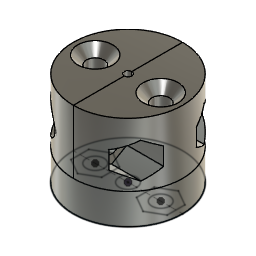
electromagnet-gripper (Autodesk Fusion 360 design; units mm, degrees)
Autodesk Fusion 360 part; units mm, degrees
note: some values were not read from the file. Chosen so that the rebuilt part matches the saved one: which bodies a step acts on; which sketch regions a step uses; which face or edge a step refers to.
sketch "Sketch1" plane through (0, 0, 0) normal (0, 0, 1) x (1, 0, 0)
sketch "Sketch1 (2)" plane through (0, 0, 0) normal (0, 0, 1) x (1, 0, 0) in component "bottom"
  circle A0 centre (0, 0) radius 12.5
  circle A1 centre (0, 0) radius 2
  circle A2 centre (-7.5, 0) radius 2
  circle A3 centre (7.5, 0) radius 2
  line L0 (0, 0) -> (12.5, 0) construction
  line L1 (0, 0) -> (-12.5, 0) construction
  line L2 (11, 2.0207) -> (7.5, 4.0415)
  line L3 (7.5, 4.0415) -> (4, 2.0207)
  line L4 (4, 2.0207) -> (4, -2.0207)
  line L5 (4, -2.0207) -> (7.5, -4.0415)
  line L6 (7.5, -4.0415) -> (11, -2.0207)
  line L7 (11, -2.0207) -> (11, 2.0207)
  line L8 (-11, -2.0207) -> (-7.5, -4.0415)
  line L9 (-7.5, -4.0415) -> (-4, -2.0207)
  line L10 (-4, -2.0207) -> (-4, 2.0207)
  line L11 (-4, 2.0207) -> (-7.5, 4.0415)
  line L12 (-7.5, 4.0415) -> (-11, 2.0207)
  line L13 (-11, 2.0207) -> (-11, -2.0207)
  point P0 (7.5, 0)
  point P1 (-7.5, 0)
  dimension "d1" = 25
  dimension "d2" = 4
  dimension "d3" = 4
  dimension "d4" = 3.5
  dimension "d6" = 5
  dimension "d7" = 5
  constraint coincident A0.centre A1.centre
  constraint horizontal L0
  constraint coincident A0 L1.end
  constraint parallel L0 L1
  constraint coincident P1 L1
  constraint equal A2 A3
  constraint coincident P0 A3.centre
  constraint coincident P1 A2.centre
  constraint equal L3 L11
  constraint vertical L10
  constraint vertical L4
  constraint coincident A0 L0.end
  constraint coincident P0 L0
  measures "d1" diameter of A0
  measures "d2" diameter of A1
  measures "d3" diameter of A3
  measures "d4" distance of P0 L7
  measures "d6" distance of A0 P1
  measures "d7" distance of A0 P0
extrude "Extrude1" add sketch "Sketch1 (2)" along normal blind 7 contours A0 | L2 L3 L4 L5 L6 L7 | L8 L9 L10 L11 L12 L13 makes body 1 in component "bottom"
extrude "Extrude2" cut sketch "Sketch1 (2)" along normal blind 3.5 contours L2 L3 L4 L5 L6 L7 | L8 L9 L10 L11 L12 L13 bodies 1 in component "bottom"
chamfer "Chamfer1" distance 2 angle 45 1 edges at (-1.8647, 0.7232, 7) on bodies 1 in component "bottom"
sketch "Sketch1 (3)" plane through (0, 0, 7) normal (0, 0, 1) x (-1, 0, 0) in component "top"
  circle A0 centre (0, 0) radius 12.5
  circle A1 centre (7.5, 0) radius 2
  circle A2 centre (-7.5, 0) radius 2
  circle A3 centre (0, 0) radius 4
  circle A4 centre (0, 0) radius 12.5
  circle A5 centre (-7.5, 0) radius 2
  circle A6 centre (7.5, 0) radius 2
extrude "Extrude1'" add sketch "Sketch1 (3)" along normal blind 14.5 separate body contours A0 A4 | A3 makes body 2 in component "top"
chamfer "Chamfer1'" distance 2 angle 45 2 edges at (-5.6353, -0.7232, 21.5) (9.3647, -0.7232, 21.5) on bodies 2 in component "top"
split "Split1" by plane through (0, 0, 0) normal (1, 0, 0) bodies 2 makes body 3 at (9.3723, 8.2711, 11.8333) in component "top"
sketch "Sketch2" plane through (0, 0, 0) normal (1, 0, 0) x (0, 1, 0) in component "top"
  line L0 (12.5, 21.5) -> (-12.5, 21.5)
  line L1 (-12.5, 21.5) -> (-12.5, 7)
  line L2 (-12.5, 7) -> (12.5, 7)
  line L3 (12.5, 7) -> (12.5, 21.5)
  line L4 (0, 21.5) -> (0, 7)
  constraint midpoint L0 L4.start
  constraint midpoint L2 L4.end
pipe "Pipe1" cut diameter 1.75 path "Sketch2" along L4 bodies 2 3 in component "top"
ref_plane "WorkPlane1" through (0, 12.5, 16.7927) normal (0, 1, 0) x (1, 0, 0) in component "top"
sketch "Sketch4" plane through (0, 0, 0) normal (0, 1, 0) x (1, 0, 0) in component "top"
  line L0 (0, -21.5) -> (0, -7)
  line L1 (0, -7) -> (0.875, -7)
  line L2 (0, -7) -> (0, -21.5)
  line L3 (0.875, -21.5) -> (0, -21.5)
  line L4 (0, -7) -> (0, -21.5)
  line L5 (0, -21.5) -> (-0.875, -21.5)
  line L6 (0, -21.5) -> (0, -7)
  line L7 (-0.875, -7) -> (0, -7)
  line L8 (0.875, -7) -> (0.875, -21.5)
  line L9 (-0.875, -21) -> (-0.875, -6.5)
  line L10 (0.875, -18.567) -> (0.625, -18.567)
  line L11 (0.625, -18.567) -> (0.875, -19)
  line L12 (0.625, -18.567) -> (1.125, -18.567) construction
  line L13 (0.875, -16.9003) -> (0.625, -16.9003)
  line L14 (0.625, -16.9003) -> (0.875, -17.3333)
  line L15 (0.875, -15.2337) -> (0.625, -15.2337)
  line L16 (0.625, -15.2337) -> (0.875, -15.6667)
  line L17 (0.875, -13.567) -> (0.625, -13.567)
  line L18 (0.625, -13.567) -> (0.875, -14)
  line L19 (0.875, -11.9003) -> (0.625, -11.9003)
  line L20 (0.625, -11.9003) -> (0.875, -12.3333)
  line L21 (0.875, -10.2337) -> (0.625, -10.2337)
  line L22 (0.625, -10.2337) -> (0.875, -10.6667)
  line L23 (0.875, -8.567) -> (0.625, -8.567)
  line L24 (0.625, -8.567) -> (0.875, -9)
  line L25 (-0.625, -13.567) -> (-0.875, -14)
  line L26 (-0.625, -15.2337) -> (-0.875, -15.6667)
  line L27 (-0.875, -16.9003) -> (-0.625, -16.9003)
  line L28 (-0.625, -18.567) -> (-0.875, -19)
  line L29 (-0.875, -11.9003) -> (-0.625, -11.9003)
  line L30 (-0.625, -16.9003) -> (-0.875, -17.3333)
  line L31 (-0.875, -8.567) -> (-0.625, -8.567)
  line L32 (-0.875, -15.2337) -> (-0.625, -15.2337)
  line L33 (-0.875, -13.567) -> (-0.625, -13.567)
  line L34 (-0.625, -10.2337) -> (-0.875, -10.6667)
  line L35 (-0.625, -11.9003) -> (-0.875, -12.3333)
  line L36 (-0.625, -18.567) -> (-1.125, -18.567) construction
  line L37 (-0.875, -7) -> (-0.875, -21.5)
  line L38 (-0.875, -10.2337) -> (-0.625, -10.2337)
  line L39 (-0.875, -18.567) -> (-0.625, -18.567)
  line L40 (-0.625, -8.567) -> (-0.875, -9)
  point P0 (-0.875, -7)
  point P1 (-0.875, -21.5)
  dimension "d23" = 0.25
  dimension "d24" = 60
  dimension "d25" = 2.5
  dimension "d28" = 0
  dimension "d29" = 10
  constraint coincident L1.end L8.start
  constraint coincident L3.start L8.end
  constraint coincident P1 L9.start
  constraint coincident P0 L9.end
  constraint coincident L8 L10.start
  constraint perpendicular L8 L10
  constraint horizontal L12
  constraint coincident L8 L11.end
  constraint symmetric L0 L1.end P0
  constraint symmetric L0 L3.start P1
  constraint symmetric L0 L10.start L39.start
  constraint symmetric L0 L10.end L28.start
  constraint symmetric L0 L11.end L28.end
  constraint symmetric L0 L12.end L36.end
  constraint symmetric L0 L13.start L27.start
  constraint symmetric L0 L13.end L27.end
  constraint symmetric L0 L14.end L30.end
  constraint symmetric L0 L15.start L32.start
  constraint symmetric L0 L15.end L26.start
  constraint symmetric L0 L16.end L26.end
  constraint symmetric L0 L17.start L33.start
  constraint symmetric L0 L17.end L25.start
  constraint symmetric L0 L18.end L25.end
  constraint symmetric L0 L19.start L29.start
  constraint symmetric L0 L19.end L29.end
  constraint symmetric L0 L20.end L35.end
  constraint symmetric L0 L21.start L38.start
  constraint symmetric L0 L21.end L34.start
  constraint symmetric L0 L22.end L34.end
  constraint symmetric L0 L23.start L31.start
  constraint symmetric L0 L23.end L31.end
  constraint symmetric L0 L24.end L40.end
  measures "d23" distance of L10.start L10.end
  measures "d24" angle of L11 L12
  measures "d25" distance of L3 L11.end
revolve "Revolve1" add sketch "Sketch4" angle 360 about axis through (0, 0, 7) along (0, 0, 1) contours L8 L10 L11 | L8 L23 L24 | L8 L13 L14 | L8 L21 L22 | L8 L15 L16 | L8 L19 L20 | L8 L17 L18 bodies 2 3 in component "top"
ref_plane "WorkPlane2" through (-12.5, 0, 14.7326) normal (-1, 0, 0) x (0, 1, 0) in component "top"
sketch "Sketch5" plane through (-12.5, 0, 0) normal (-1, 0, 0) x (0, -1, 0) in component "top"
  line L0 (-2, 19.5) -> (2, 19.5)
  line L1 (4, 21.5) -> (-4, 21.5)
  circle A0 centre (-7.25, 13) radius 2
  circle A1 centre (7.25, 13) radius 2
  line L2 (12.5, 21.5) -> (-12.5, 21.5)
  line L3 (12.5, 7) -> (-12.5, 7)
  line L4 (-12.5, 21.5) -> (-12.5, 7) construction
  circle A2 centre (-7.25, 13) radius 4
  circle A3 centre (7.25, 13) radius 4
  line L5 (-2, 19.5) -> (-2, 14.25) construction
  line L6 (-2, 14.25) -> (-12.5, 14.25) construction
  line L7 (2, 19.5) -> (2, 13) construction
  line L8 (2, 13) -> (12.5, 13) construction
  dimension "d32" = 4
  dimension "d33" = 4
  dimension "d34" = 8
  dimension "d35" = 8
  constraint coincident L2.end L4.start
  constraint coincident L3.end L4.end
  constraint concentric A0 A2
  constraint concentric A1 A3
  constraint coincident L0.start L5.start
  constraint midpoint L4 L6.end
  constraint perpendicular L4 L6
  constraint coincident L0.end L7.start
  constraint perpendicular L7 L8
  measures "d32" diameter of A0
  measures "d33" diameter of A1
  measures "d34" diameter of A2
  measures "d35" diameter of A3
extrude "Extrude2'" cut sketch "Sketch5" against normal blind 25 contours A0 | A1 bodies 2 in component "top"
extrude "Extrude3" cut sketch "Sketch5" against normal blind 7.5 bodies 2 in component "top"
chamfer "Chamfer2" distance 2 angle 45 1 edges at (-5, 9.1147, 12.2768) on bodies 2 in component "top"
chamfer "Chamfer2" distance 2 angle 45 1 edges at (-5, -5.3853, 12.2768) on bodies 2 in component "top"
ref_plane "WorkPlane3" through (12.5, 0, 12.6325) normal (1, 0, 0) x (0, -1, 0) in component "top"
sketch "Sketch6" plane through (12.5, 0, 0) normal (1, 0, 0) x (0, 1, 0) in component "top"
  spline S0 degree 3 poles (-5.25, 13) (-5.25, 12.7522) (-5.2991, 12.4895) (-5.4927, 12.0107) (-5.6371, 11.7947) (-5.9895, 11.4222) (-6.2304, 11.2575) (-6.7398, 11.0466) (-7.0079, 11) (-7.5214, 11) (-7.8042, 11.0577) (-8.3204, 11.2871) (-8.5541, 11.4582) (-8.8822, 11.8248) (-9.0148, 12.027) (-9.1529, 12.372) (-9.1891, 12.494) (-9.2377, 12.7444) (-9.25, 12.8729) (-9.25, 13.1271) (-9.2377, 13.2556) (-9.1891, 13.506) (-9.1529, 13.628) (-9.0148, 13.973) (-8.8822, 14.1752) (-8.5541, 14.5418) (-8.3204, 14.7129) (-7.8042, 14.9423) (-7.5214, 15) (-7.0079, 15) (-6.7398, 14.9534) (-6.2304, 14.7425) (-5.9895, 14.5778) (-5.6371, 14.2053) (-5.4927, 13.9893) (-5.2991, 13.5105) (-5.25, 13.2478) (-5.25, 13) knots 0 0 0 0 0.074346 0.074346 0.148693 0.148693 0.237845 0.237845 0.326997 0.326997 0.426948 0.426948 0.526899 0.526899 0.603159 0.603159 0.64129 0.64129 0.67942 0.67942 0.71755 0.71755 0.75568 0.75568 0.83194 0.83194 0.931892 0.931892 1.031843 1.031843 1.120995 1.120995 1.210146 1.210146 1.284493 1.284493 1.358839 1.358839 1.358839 1.358839
  spline S1 degree 3 poles (9.25, 13) (9.25, 12.8729) (9.2377, 12.7444) (9.1891, 12.494) (9.1529, 12.372) (9.0148, 12.027) (8.8822, 11.8248) (8.5541, 11.4582) (8.3204, 11.2871) (7.8042, 11.0577) (7.5214, 11) (7.0079, 11) (6.7398, 11.0466) (6.2304, 11.2575) (5.9895, 11.4222) (5.6371, 11.7947) (5.4927, 12.0107) (5.2991, 12.4895) (5.25, 12.7522) (5.25, 13.2478) (5.2991, 13.5105) (5.4927, 13.9893) (5.6371, 14.2053) (5.9895, 14.5778) (6.2304, 14.7425) (6.7398, 14.9534) (7.0079, 15) (7.5214, 15) (7.8042, 14.9423) (8.3204, 14.7129) (8.5541, 14.5418) (8.8822, 14.1752) (9.0148, 13.973) (9.1529, 13.628) (9.1891, 13.506) (9.2377, 13.2556) (9.25, 13.1271) (9.25, 13) knots 0 0 0 0 0.03813 0.03813 0.07626 0.07626 0.152521 0.152521 0.252472 0.252472 0.352423 0.352423 0.441575 0.441575 0.530727 0.530727 0.605073 0.605073 0.67942 0.67942 0.753766 0.753766 0.828113 0.828113 0.917264 0.917264 1.006416 1.006416 1.106367 1.106367 1.206319 1.206319 1.282579 1.282579 1.320709 1.320709 1.358839 1.358839 1.358839 1.358839
  line L0 (-5.25, 13) -> (-9.25, 13) construction
  line L1 (-3.75, 15.0207) -> (-7.25, 17.0415)
  line L2 (-7.25, 17.0415) -> (-10.75, 15.0207)
  line L3 (-10.75, 15.0207) -> (-10.75, 10.9793)
  line L4 (-10.75, 10.9793) -> (-7.25, 8.9585)
  line L5 (-7.25, 8.9585) -> (-3.75, 10.9793)
  line L6 (-3.75, 10.9793) -> (-3.75, 15.0207)
  line L7 (0, 7) -> (0, 21.5)
  line L8 (3.75, 15.0207) -> (7.25, 17.0415)
  line L9 (7.25, 17.0415) -> (10.75, 15.0207)
  line L10 (10.75, 15.0207) -> (10.75, 10.9793)
  line L11 (10.75, 10.9793) -> (7.25, 8.9585)
  line L12 (7.25, 8.9585) -> (3.75, 10.9793)
  line L13 (3.75, 10.9793) -> (3.75, 15.0207)
  point P0 (-7.25, 13)
  dimension "d43" = 3.5
  constraint coincident S0.start S0.end
  constraint coincident S0 L0.end
  constraint horizontal L0
  constraint midpoint L0 P0
  constraint symmetric L1.start L7 L8.start
  constraint symmetric L1.end L7 L8.end
  constraint symmetric L2.end L7 L9.end
  constraint symmetric L3.end L7 L10.end
  constraint symmetric L4.end L7 L11.end
  constraint symmetric L5.end L7 L12.end
  measures "d43" distance of P0 L6
extrude "Extrude4" cut sketch "Sketch6" against normal blind 9 contours S0 | S1 | L1 L2 L3 L4 L5 L6 | L8 L9 L10 L11 L12 L13 bodies 2 in component "top"
split "Split2" by plane through (0, 0, 0) normal (1, 0, 0) bodies 2 makes body 4 at (4.613, 11.6177, 14.5069) in component "top"
component "bottom" placed x (1, 0, 0) y (0, 1, 0) z (0, 0, 1) at (0, 0, 0)
component "top" placed x (1, 0, 0) y (0, 1, 0) z (0, 0, 1) at (0, 0, 0)
